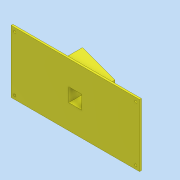
# Autodesk Inventor part: touchscreen_support
Saved by Autodesk Inventor 2022 (Build 260153000, 153)
## iProperties
Created: 2020-11-06
Part Number: touchscreen_support
Material: Generic
Document SubType Name: Modeling
Designer: nnico
Density: 1 g/cm^3
Appearance: Yellow
Author: nnico
Autodesk Inventor part; units mm, degrees
ref_plane "YZ Plane" through (0, 0, 0) normal (1, 0, 0) x (0, 1, 0)
ref_plane "XZ Plane" through (0, 0, 0) normal (0, 1, 0) x (-1, 0, 0)
ref_plane "XY Plane" through (0, 0, 0) normal (0, 0, 1) x (1, 0, 0)
sketch "Sketch1" plane through (0, 0, 0) normal (0, 1, 0) x (-1, 0, 0)
  line L0 (70, 34) -> (-70, 34)
  line L1 (-70, 34) -> (-70, -34)
  line L2 (-70, -34) -> (70, -34)
  line L3 (70, -34) -> (70, 34)
  line L4 (70, 0) -> (-70, 0) construction
  line L5 (0, 34) -> (0, -34) construction
  line L6 (70, 34) -> (66, 34) construction
  line L7 (66, 34) -> (66, 30) construction
  line L8 (66, 30) -> (70, 30) construction
  line L9 (70, 30) -> (70, 34) construction
  circle A0 centre (66, 30) radius 1.25
  circle A1 centre (66, -30) radius 1.25
  circle A2 centre (-66, 30) radius 1.25
  circle A3 centre (-66, -30) radius 1.25
  point P0 (0, 0)
  point P1 (0, 0)
  dimension "d0" = 68
  dimension "d1" = 140
  dimension "d4" = 4
  dimension "d5" = 4
  dimension "d6" = 2.5
  constraints: 20 end point, 5 midpoint, 4 centre point, 4 parallel, 3 symmetric about line, 2 coincident, 2 horizontal, 2 perpendicular, 3 other
  measures "d0" distance of L2.end L0.start
  measures "d1" distance of L0.start L0.end
  measures "d4" distance of L8.end L7.end
  measures "d5" distance of L7.end L6.end
  measures "d6" diameter of A0
extrude "Extrusion1" add sketch "Sketch1" along normal blind 2
sketch "Sketch2" plane through (0, 2, 0) normal (0, 1, 0) x (1, 0, 0)
  line L0 (-24.1481, -20) -> (24.1481, -20)
  line L1 (24.1481, -20) -> (24.1481, 20)
  line L2 (24.1481, 20) -> (-24.1481, 20)
  line L3 (-24.1481, 20) -> (-24.1481, -20)
  line L4 (-24.1481, 0) -> (24.1481, 0) construction
  line L5 (0, -20) -> (0, 20) construction
  point P0 (0, 0)
  point P1 (0, 0)
  dimension "d7" = 48.2963
  dimension "d8" = 40
  constraints: 12 end point, 5 midpoint, 2 parallel, 1 coincident, 1 horizontal, 1 perpendicular
  measures "d7" distance of L2.end L1.end
  measures "d8" distance of L1.end L0.end
extrude "Extrusion2" add sketch "Sketch2" along normal blind 30
sketch "Sketch3" plane through (-24.1481, 2, 20) normal (0, 0, 1) x (1, 0, 0)
  line L0 (0, 0) -> (0, 30) projected
  line L1 (0, 30) -> (48.2963, 17.059)
  line L2 (48.2963, 0) -> (48.2963, 30) projected
  line L3 (0, 30) -> (48.2963, 30) projected
  point P0 (24.1481, -2)
  dimension "d11" = 15
  constraints: 2 end point, 1 point on line
  measures "d11" angle of L3 L1
extrude "Extrusion3" cut sketch "Sketch3" against normal up to next
sketch "Sketch5" plane through (-24.1481, 32, 20) normal (0.2588, 0.9659, 0) x (0.9659, -0.2588, 0)
  line L0 (40, 5) -> (10, 5) construction
  line L1 (10, 5) -> (10, 35) construction
  line L2 (10, 35) -> (40, 35) construction
  line L3 (40, 35) -> (40, 5) construction
  line L4 (50, 40) -> (50, 0) construction
  line L5 (50, 20) -> (0, 20) construction
  line L6 (0, 40) -> (0, 0) construction
  line L7 (7.7646, 40) -> (0, 40) construction
  line L8 (7.7646, 0) -> (0, 0) construction
  line L9 (40, 20) -> (10, 20) construction
  circle A0 centre (40, 5) radius 2.5
  circle A1 centre (40, 35) radius 2.5
  circle A2 centre (10, 35) radius 2.5
  circle A3 centre (10, 5) radius 2.5
  point P0 (31.6075, 20)
  point P1 (25, 20)
  dimension "d18" = 30
  dimension "d19" = 30
  dimension "d20" = 5
  dimension "d21" = 5
  dimension "d22" = 5
  dimension "d23" = 5
  constraints: 12 end point, 6 midpoint, 4 centre point, 4 coincident, 2 parallel, 1 horizontal, 1 perpendicular
  measures "d18" distance of L1.end L2.end
  measures "d19" distance of L0.end L1.end
  measures "d20" diameter of A0
  measures "d21" diameter of A1
  measures "d22" diameter of A2
  measures "d23" diameter of A3
extrude "Extrusion5" cut sketch "Sketch5" against normal blind 7
sketch "Sketch6" plane through (0, 0, 0) normal (0, -1, 0) x (1, 0, 0)
  line L0 (-24.1481, -20) -> (24.1481, -20) projected
  line L1 (24.1481, -20) -> (24.1481, 20) projected
  line L2 (-24.1481, 20) -> (-24.1481, -20) projected
  line L3 (24.1481, 20) -> (-24.1481, 20) projected
  line L4 (-7.2444, 7.5) -> (7.2444, 7.5)
  line L5 (7.2444, 7.5) -> (7.2444, -7.5)
  line L6 (7.2444, -7.5) -> (-7.2444, -7.5)
  line L7 (-7.2444, -7.5) -> (-7.2444, 7.5)
  line L8 (0, -7.5) -> (0, 7.5) construction
  point P0 (0, 0)
  point P1 (0, 0)
  dimension "d26" = 14.4889
  dimension "d27" = 15
  constraints: 10 end point, 3 midpoint, 2 parallel, 1 coincident, 1 horizontal, 1 perpendicular
  measures "d26" distance of L5.end L6.end
  measures "d27" distance of L4.end L5.end
extrude "Extrusion6" cut sketch "Sketch6" against normal up to next contours L4 L5 L6 L7
body "Solid1"
